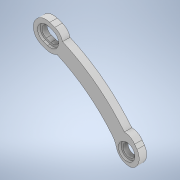
# Autodesk Inventor part: Part3
Saved by Autodesk Inventor 2020.3 (Build 243373000, 373)
## iProperties
Created: 2019-08-12
Part Number: Part3
Material: Generic
Document SubType Name: Modeling
Designer: Horváth Patrik
Density: 1 g/cm^3
Appearance: Default
Author: Horváth Patrik
Autodesk Inventor part; units mm, degrees
ref_plane "YZ Plane" through (0, 0, 0) normal (1, 0, 0) x (0, 1, 0)
ref_plane "XZ Plane" through (0, 0, 0) normal (0, 1, 0) x (-1, 0, 0)
ref_plane "XY Plane" through (0, 0, 0) normal (0, 0, 1) x (1, 0, 0)
ref_plane "Work Plane1" through (37.0364, -24.4328, 1) normal (0, 0, 1) x (1, 0, 0)
sketch "Sketch2" plane through (37.0364, -24.4328, 1) normal (0, 0, 1) x (1, 0, 0)
  circle A0 centre (0, 0) radius 3 construction
  circle A1 centre (0, 0) radius 1.25 projected
  circle A2 centre (-31.5364, 24.4328) radius 3 construction
  circle A3 centre (-31.5364, 24.4328) radius 1.4795 projected
  circle A4 centre (0, 0) radius 1.25 projected
  circle A5 centre (-31.5364, 24.4328) radius 1.4795 projected
  arc A6 (0, 0) -> (-31.5364, 24.4328) centre (-52.3674, -35.0237) ccw construction
  arc A7 (2.4937, 1.6678) -> (-30.5445, 27.264) centre (-52.3674, -35.0237) ccw
  arc A8 (-2.4937, -1.6678) -> (-32.5284, 21.6015) centre (-52.3674, -35.0237) ccw
  arc A9 (-2.4937, -1.6678) -> (2.4937, 1.6678) centre (0, 0) ccw
  arc A10 (-30.5445, 27.264) -> (-32.5284, 21.6015) centre (-31.5364, 24.4328) ccw
  point P0 (-37.0364, 24.4328)
  dimension "d3" = 60
  constraints: 10 point on circle, 5 centre point, 4 tangent, 1 concentric
  measures "d3" radius of A8
extrude "Extrusion2" add sketch "Sketch2" along normal blind 3
sketch "Sketch4" plane through (5.5, 0, 4) normal (0, 0, 1) x (1, 0, 0)
  arc A0 (29.0427, -26.1006) -> (-0.992, -2.8313) centre (-20.831, -59.4565) ccw construction
  arc A1 (34.0301, -22.765) -> (0.992, 2.8313) centre (-20.831, -59.4565) ccw construction
  circle A2 centre (0, 0) radius 3 construction
  circle A3 centre (0, 0) radius 1.4795 construction
  arc A4 (0.9411, -0.3381) -> (-0.9463, 0.3231) centre (-20.831, -59.4565) ccw construction
  arc A5 (2.669, 4.3538) -> (0.6318, 5.0676) centre (-20.831, -59.4565) ccw
  arc A6 (-0.7868, -5.0301) -> (-2.5245, -4.4213) centre (-20.831, -59.4565) ccw
  arc A7 (-0.7868, -5.0301) -> (2.669, 4.3538) centre (0.9411, -0.3381) ccw
  arc A8 (0.6318, 5.0676) -> (-2.5245, -4.4213) centre (-0.9463, 0.3231) ccw
  arc A9 (0.992, 2.8313) -> (-0.992, -2.8313) centre (0, 0) ccw projected
  arc A10 (29.0427, -26.1006) -> (34.0301, -22.765) centre (31.5364, -24.4328) ccw projected
  dimension "d15" = 10
  dimension "d30" = 1
  dimension "d31" = 1
  constraints: 11 point on circle, 5 centre point, 4 tangent, 1 coincident, 1 concentric
  measures "d15" radial gap between concentric circles of A6 A5
  measures "d30" distance of A4.end point (0, 0)
  measures "d31" distance of point (0, 0) A4.start
extrude "Extrusion4" add sketch "Sketch4" against normal blind 3
sketch "Sketch5" plane through (37.0364, -24.4328, 4) normal (0, 0, 1) x (1, 0, 0)
  arc A0 (-30.5953, 24.0947) -> (-32.4828, 24.7559) centre (-52.3674, -35.0237) ccw construction
  arc A1 (-29.7313, 26.4406) -> (-31.6937, 27.1281) centre (-52.3674, -35.0237) ccw
  arc A2 (-31.4593, 21.7487) -> (-33.2718, 22.3837) centre (-52.3674, -35.0237) ccw
  arc A3 (-31.4593, 21.7487) -> (-29.7313, 26.4406) centre (-30.5953, 24.0947) ccw
  arc A4 (-31.6937, 27.1281) -> (-33.2718, 22.3837) centre (-32.4828, 24.7559) ccw
  arc A5 (-30.9046, 29.5004) -> (-34.0609, 20.0115) centre (-32.4828, 24.7559) ccw projected
  arc A6 (-32.3233, 19.4027) -> (-34.0609, 20.0115) centre (-52.3674, -35.0237) ccw projected
  arc A7 (-28.8674, 28.7866) -> (-30.9046, 29.5004) centre (-52.3674, -35.0237) ccw projected
  arc A8 (-25.7624, 25.3765) -> (-28.8674, 28.7866) centre (-30.5953, 24.0947) ccw projected
  arc A9 (-32.3233, 19.4027) -> (-28.0148, 19.812) centre (-30.5953, 24.0947) ccw projected
  arc A10 (-29.4549, 27.1913) -> (-31.4412, 27.8873) centre (-52.3674, -35.0237) ccw
  arc A11 (-31.4412, 27.8873) -> (-33.5243, 21.6246) centre (-32.4828, 24.7559) ccw
  arc A12 (-31.7358, 20.998) -> (-33.5243, 21.6246) centre (-52.3674, -35.0237) ccw
  arc A13 (-31.7358, 20.998) -> (-29.4549, 27.1913) centre (-30.5953, 24.0947) ccw
  dimension "d18" = 5
  dimension "d35" = 0.8
  constraints: 18 point on circle, 9 centre point, 4 tangent, 2 coincident, 2 concentric, 3 other
  measures "d18" radial gap between concentric circles of A2 A1
  measures "d35" radial gap between concentric circles of A3 A13
extrude "Extrusion5" cut sketch "Sketch5" against normal blind 5 contours A3 A2 A4 A1
sketch "Sketch6" plane through (37.0364, -24.4328, 1) normal (0, 0, -1) x (-1, 0, 0)
  circle A0 centre (0, 0) radius 1.25 projected
  circle A1 centre (0, 0) radius 2.5
  arc A2 (-4.1194, 2.8338) -> (4.1194, -2.8338) centre (0, 0) ccw
  arc A3 (31.5364, 24.4328) -> (0, 0) centre (52.3674, -35.0237) ccw construction
  arc A4 (5.0542, -1.475) -> (-3.1846, 4.1926) centre (0.9348, 1.3588) ccw
  line L0 (-4.1194, 2.8338) -> (-3.1846, 4.1926)
  line L1 (4.1194, -2.8338) -> (5.0542, -1.475)
  line L2 (-0.7345, 0.4913) -> (0.6872, -0.4596) construction
  line L3 (1.7213, 0.8024) -> (-0.0122, 2.0287) construction
  circle A5 centre (0, 0) radius 3.3
  point P0 (37.0364, 24.4328)
  dimension "d19" = 5
  dimension "d22" = 10
  dimension "d29" = 1.5
  dimension "d32" = 6.6
  constraints: 8 end point, 5 point on circle, 4 centre point, 4 tangent, 3 coincident, 2 line through centre, 2 point on line, 1 equal radius
  measures "d19" diameter of A1
  measures "d22" diameter of A2
  measures "d29" angle of L2 L3
  measures "d32" diameter of A5
extrude "Extrusion6" cut sketch "Sketch6" against normal up to surface (3 mm away) contours A1
extrude "Extrusion7" add sketch "Sketch6" against normal up to surface (3 mm away) contours L0 A4 L1 A2 | A5
sketch "Sketch7" plane through (37.0364, -24.4328, 4) normal (0, 0, 1) x (1, 0, 0)
  circle A0 centre (0, 0) radius 3.3 projected
  point P0 (-37.0364, 24.4328)
extrude "Extrusion8" cut sketch "Sketch7" against normal blind 1
extrude "Extrusion9" cut sketch "Sketch5" against normal blind 1
sketch "Sketch8" plane through (37.0364, -24.4328, 4) normal (0, 0, 1) x (1, 0, 0)
  arc A0 (-4.1194, -2.8338) -> (4.1194, 2.8338) centre (0, 0) ccw projected
  arc A1 (-4.1466, -0.5304) -> (2.2951, -4.4421) centre (0.9806, 0.653) ccw
  arc A2 (-5.7407, 2.7382) -> (-28.0148, 19.812) centre (-52.3674, -35.0237) ccw projected
  arc A3 (-4.1466, -0.5304) -> (-5.7407, 2.7382) centre (-12.0206, -2.3478) ccw
  arc A4 (-31.4412, 27.8873) -> (-33.5243, 21.6246) centre (-32.4828, 24.7559) ccw projected
  arc A5 (-29.4549, 27.1913) -> (-31.4412, 27.8873) centre (-52.3674, -35.0237) ccw projected
  arc A6 (-31.7358, 20.998) -> (-29.4549, 27.1913) centre (-30.5953, 24.0947) ccw projected
  arc A7 (-31.7358, 20.998) -> (-33.5243, 21.6246) centre (-52.3674, -35.0237) ccw projected
  circle A8 centre (0, 0) radius 3.3 projected
  arc A9 (-0.9525, 6.3588) -> (-25.7624, 25.3765) centre (-52.3674, -35.0237) ccw projected
  arc A10 (-25.7624, 25.3765) -> (-28.8674, 28.7866) centre (-30.5953, 24.0947) ccw projected
  arc A11 (-28.8674, 28.7866) -> (-30.9046, 29.5004) centre (-52.3674, -35.0237) ccw projected
  arc A12 (-30.9046, 29.5004) -> (-34.0609, 20.0115) centre (-32.4828, 24.7559) ccw projected
  arc A13 (-32.3233, 19.4027) -> (-34.0609, 20.0115) centre (-52.3674, -35.0237) ccw projected
  arc A14 (-32.3233, 19.4027) -> (-28.0148, 19.812) centre (-30.5953, 24.0947) ccw projected
  arc A15 (-5.7407, 2.7382) -> (-28.0148, 19.812) centre (-52.3674, -35.0237) ccw projected
  arc A16 (-5.7407, 2.7382) -> (-5.0542, -1.475) centre (-0.9348, 1.3588) ccw projected
  line L0 (-4.1194, -2.8338) -> (-5.0542, -1.475) projected
  arc A17 (-4.1194, -2.8338) -> (4.1194, 2.8338) centre (0, 0) ccw projected
  line L1 (3.1846, 4.1926) -> (4.1194, 2.8338) projected
  arc A18 (3.1846, 4.1926) -> (-0.9525, 6.3588) centre (-0.9348, 1.3588) ccw projected
  point P0 (-37.0364, 24.4328)
  constraints: 7 point on circle, 2 centre point, 2 tangent
extrude "Extrusion10" cut sketch "Sketch8" against normal up to surface (3 mm away) contours L0 A16 A3 A1 A0
fillet "Fillet1" radius 3 1 edges at (39.3315, -28.8749, 2.5)
body "Solid1"
